Autodesk Inventor part; units mm, degrees
(part 4 of 4)
  line L1499 (-9.3571, 29.0765) -> (-9.424, 29.0765) construction
  spline S459 degree 2 poles (-9.424, 29.0765) (-9.4797, 29.0765) (-9.5645, 29.1568) (-9.5645, 29.2103) knots 0 0 0 1 2 2 2
  line L1500 (-9.424, 29.0765) -> (-9.4797, 29.0765) construction
  line L1501 (-9.4797, 29.0765) -> (-9.5645, 29.1568) construction
  line L1502 (-9.5645, 29.1568) -> (-9.5645, 29.2103) construction
  spline S460 degree 2 poles (-9.5645, 29.2103) (-9.5645, 29.2505) (-9.54, 29.2862) knots 0 0 0 1 1 1
  line L1503 (-9.5645, 29.2103) -> (-9.5645, 29.2505) construction
  line L1504 (-9.5645, 29.2505) -> (-9.54, 29.2862) construction
  line L1505 (-9.54, 29.2862) -> (-9.1385, 29.8883)
  spline S461 degree 2 poles (-9.1385, 29.8883) (-9.3392, 29.9218) (-9.4574, 30.0801) knots 0 0 0 1 1 1
  line L1506 (-9.1385, 29.8883) -> (-9.3392, 29.9218) construction
  line L1507 (-9.3392, 29.9218) -> (-9.4574, 30.0801) construction
  spline S462 degree 2 poles (-9.4574, 30.0801) (-9.5623, 30.2229) (-9.5623, 30.4147) knots 0 0 0 1 1 1
  line L1508 (-9.4574, 30.0801) -> (-9.5623, 30.2229) construction
  line L1509 (-9.5623, 30.2229) -> (-9.5623, 30.4147) construction
  spline S463 degree 2 poles (-9.5623, 30.4147) (-9.5623, 30.631) (-9.4284, 30.7804) knots 0 0 0 1 1 1
  line L1510 (-9.5623, 30.4147) -> (-9.5623, 30.631) construction
  line L1511 (-9.5623, 30.631) -> (-9.4284, 30.7804) construction
  spline S464 degree 2 poles (-9.4284, 30.7804) (-9.2812, 30.9477) (-9.0292, 30.9477) knots 0 0 0 1 1 1
  line L1512 (-9.4284, 30.7804) -> (-9.2812, 30.9477) construction
  line L1513 (-9.2812, 30.9477) -> (-9.0292, 30.9477) construction
  line L1514 (-9.0292, 30.9477) -> (-8.3624, 30.9477)
  spline S465 degree 2 poles (-8.3624, 30.9477) (-8.2285, 30.9477) (-8.2285, 30.8139) knots 0 0 0 1 1 1
  line L1515 (-8.3624, 30.9477) -> (-8.2285, 30.9477) construction
  line L1516 (-8.2285, 30.9477) -> (-8.2285, 30.8139) construction
  line L1517 (-8.2285, 30.8139) -> (-8.2285, 29.2126)
  spline S466 degree 2 poles (-8.2285, 29.2126) (-8.2285, 29.0787) (-8.3624, 29.0787) knots 0 0 0 1 1 1
  line L1518 (-8.2285, 29.2126) -> (-8.2285, 29.0787) construction
  line L1519 (-8.2285, 29.0787) -> (-8.3624, 29.0787) construction
  spline S467 degree 2 poles (-8.3624, 29.0787) (-8.4962, 29.0787) (-8.4962, 29.2126) knots 0 0 0 1 1 1
  line L1520 (-8.3624, 29.0787) -> (-8.4962, 29.0787) construction
  line L1521 (-8.4962, 29.0787) -> (-8.4962, 29.2126) construction
  spline S468 degree 2 poles (-7.1602, 29.8794) (-7.2941, 29.8794) (-7.2941, 30.0132) knots 0 0 0 1 1 1
  line L1522 (-7.1602, 29.8794) -> (-7.2941, 29.8794) construction
  line L1523 (-7.2941, 29.8794) -> (-7.2941, 30.0132) construction
  spline S469 degree 2 poles (-7.2941, 30.0132) (-7.2941, 30.147) (-7.1602, 30.147) knots 0 0 0 1 1 1
  line L1524 (-7.2941, 30.0132) -> (-7.2941, 30.147) construction
  line L1525 (-7.2941, 30.147) -> (-7.1602, 30.147) construction
  line L1526 (-7.1602, 30.147) -> (-7.0264, 30.147)
  spline S470 degree 2 poles (-7.0264, 30.147) (-6.9015, 30.147) (-6.8279, 30.2296) knots 0 0 0 1 1 1
  line L1527 (-7.0264, 30.147) -> (-6.9015, 30.147) construction
  line L1528 (-6.9015, 30.147) -> (-6.8279, 30.2296) construction
  spline S471 degree 2 poles (-6.8279, 30.2296) (-6.761, 30.3054) (-6.761, 30.4147) knots 0 0 0 1 1 1
  line L1529 (-6.8279, 30.2296) -> (-6.761, 30.3054) construction
  line L1530 (-6.761, 30.3054) -> (-6.761, 30.4147) construction
  spline S472 degree 2 poles (-6.761, 30.4147) (-6.761, 30.524) (-6.8279, 30.5976) knots 0 0 0 1 1 1
  line L1531 (-6.761, 30.4147) -> (-6.761, 30.524) construction
  line L1532 (-6.761, 30.524) -> (-6.8279, 30.5976) construction
  spline S473 degree 2 poles (-6.8279, 30.5976) (-6.9015, 30.6801) (-7.0287, 30.6801) knots 0 0 0 1 1 1
  line L1533 (-6.8279, 30.5976) -> (-6.9015, 30.6801) construction
  line L1534 (-6.9015, 30.6801) -> (-7.0287, 30.6801) construction
  line L1535 (-7.0287, 30.6801) -> (-7.1625, 30.6801)
  spline S474 degree 2 poles (-7.1625, 30.6801) (-7.3431, 30.6801) (-7.4814, 30.573) knots 0 0 0 1 1 1
  line L1536 (-7.1625, 30.6801) -> (-7.3431, 30.6801) construction
  line L1537 (-7.3431, 30.6801) -> (-7.4814, 30.573) construction
  spline S475 degree 2 poles (-7.4814, 30.573) (-7.5215, 30.544) (-7.5639, 30.544) knots 0 0 0 1 1 1
  line L1538 (-7.4814, 30.573) -> (-7.5215, 30.544) construction
  line L1539 (-7.5215, 30.544) -> (-7.5639, 30.544) construction
  spline S476 degree 2 poles (-7.5639, 30.544) (-7.6175, 30.544) (-7.6977, 30.6266) (-7.6977, 30.6823) knots 0 0 0 1 2 2 2
  line L1540 (-7.5639, 30.544) -> (-7.6175, 30.544) construction
  line L1541 (-7.6175, 30.544) -> (-7.6977, 30.6266) construction
  line L1542 (-7.6977, 30.6266) -> (-7.6977, 30.6823) construction
  spline S477 degree 2 poles (-7.6977, 30.6823) (-7.6977, 30.7448) (-7.642, 30.7871) knots 0 0 0 1 1 1
  line L1543 (-7.6977, 30.6823) -> (-7.6977, 30.7448) construction
  line L1544 (-7.6977, 30.7448) -> (-7.642, 30.7871) construction
  spline S478 degree 2 poles (-7.642, 30.7871) (-7.4346, 30.9477) (-7.1625, 30.9477) knots 0 0 0 1 1 1
  line L1545 (-7.642, 30.7871) -> (-7.4346, 30.9477) construction
  line L1546 (-7.4346, 30.9477) -> (-7.1625, 30.9477) construction
  line L1547 (-7.1625, 30.9477) -> (-7.0287, 30.9477)
  spline S479 degree 2 poles (-7.0287, 30.9477) (-6.7766, 30.9477) (-6.6272, 30.7827) knots 0 0 0 1 1 1
  line L1548 (-7.0287, 30.9477) -> (-6.7766, 30.9477) construction
  line L1549 (-6.7766, 30.9477) -> (-6.6272, 30.7827) construction
  spline S480 degree 2 poles (-6.6272, 30.7827) (-6.4934, 30.631) (-6.4934, 30.4147) knots 0 0 0 1 1 1
  line L1550 (-6.6272, 30.7827) -> (-6.4934, 30.631) construction
  line L1551 (-6.4934, 30.631) -> (-6.4934, 30.4147) construction
  spline S481 degree 2 poles (-6.4934, 30.4147) (-6.4934, 30.1671) (-6.6607, 30.0132) knots 0 0 0 1 1 1
  line L1552 (-6.4934, 30.4147) -> (-6.4934, 30.1671) construction
  line L1553 (-6.4934, 30.1671) -> (-6.6607, 30.0132) construction
  spline S482 degree 2 poles (-6.6607, 30.0132) (-6.4934, 29.8593) (-6.4934, 29.6118) knots 0 0 0 1 1 1
  line L1554 (-6.6607, 30.0132) -> (-6.4934, 29.8593) construction
  line L1555 (-6.4934, 29.8593) -> (-6.4934, 29.6118) construction
  spline S483 degree 2 poles (-6.4934, 29.6118) (-6.4934, 29.3932) (-6.6272, 29.2438) knots 0 0 0 1 1 1
  line L1556 (-6.4934, 29.6118) -> (-6.4934, 29.3932) construction
  line L1557 (-6.4934, 29.3932) -> (-6.6272, 29.2438) construction
  spline S484 degree 2 poles (-6.6272, 29.2438) (-6.7766, 29.0787) (-7.0287, 29.0787) knots 0 0 0 1 1 1
  line L1558 (-6.6272, 29.2438) -> (-6.7766, 29.0787) construction
  line L1559 (-6.7766, 29.0787) -> (-7.0287, 29.0787) construction
  line L1560 (-7.0287, 29.0787) -> (-7.1625, 29.0787)
  spline S485 degree 2 poles (-7.1625, 29.0787) (-7.4346, 29.0787) (-7.642, 29.2393) knots 0 0 0 1 1 1
  line L1561 (-7.1625, 29.0787) -> (-7.4346, 29.0787) construction
  line L1562 (-7.4346, 29.0787) -> (-7.642, 29.2393) construction
  spline S486 degree 2 poles (-7.642, 29.2393) (-7.6977, 29.2817) (-7.6977, 29.3441) knots 0 0 0 1 1 1
  line L1563 (-7.642, 29.2393) -> (-7.6977, 29.2817) construction
  line L1564 (-7.6977, 29.2817) -> (-7.6977, 29.3441) construction
  spline S487 degree 2 poles (-7.6977, 29.3441) (-7.6977, 29.3999) (-7.6175, 29.4824) (-7.5639, 29.4824) knots 0 0 0 1 2 2 2
  line L1565 (-7.6977, 29.3441) -> (-7.6977, 29.3999) construction
  line L1566 (-7.6977, 29.3999) -> (-7.6175, 29.4824) construction
  line L1567 (-7.6175, 29.4824) -> (-7.5639, 29.4824) construction
  spline S488 degree 2 poles (-7.5639, 29.4824) (-7.5215, 29.4824) (-7.4814, 29.4534) knots 0 0 0 1 1 1
  line L1568 (-7.5639, 29.4824) -> (-7.5215, 29.4824) construction
  line L1569 (-7.5215, 29.4824) -> (-7.4814, 29.4534) construction
  spline S489 degree 2 poles (-7.4814, 29.4534) (-7.3431, 29.3464) (-7.1625, 29.3464) knots 0 0 0 1 1 1
  line L1570 (-7.4814, 29.4534) -> (-7.3431, 29.3464) construction
  line L1571 (-7.3431, 29.3464) -> (-7.1625, 29.3464) construction
  line L1572 (-7.1625, 29.3464) -> (-7.0287, 29.3464)
  spline S490 degree 2 poles (-7.0287, 29.3464) (-6.9015, 29.3464) (-6.8279, 29.4311) knots 0 0 0 1 1 1
  line L1573 (-7.0287, 29.3464) -> (-6.9015, 29.3464) construction
  line L1574 (-6.9015, 29.3464) -> (-6.8279, 29.4311) construction
  spline S491 degree 2 poles (-6.8279, 29.4311) (-6.761, 29.5069) (-6.761, 29.6162) knots 0 0 0 1 1 1
  line L1575 (-6.8279, 29.4311) -> (-6.761, 29.5069) construction
  line L1576 (-6.761, 29.5069) -> (-6.761, 29.6162) construction
  spline S492 degree 2 poles (-6.761, 29.6162) (-6.761, 29.8549) (-6.993, 29.8794) knots 0 0 0 1 1 1
  line L1577 (-6.761, 29.6162) -> (-6.761, 29.8549) construction
  line L1578 (-6.761, 29.8549) -> (-6.993, 29.8794) construction
  line L1579 (-6.993, 29.8794) -> (-7.1602, 29.8794)
  circle A34 centre (12.0262, -0.3274) radius 1.5
  circle A35 centre (7.9565, 12.6117) radius 1.5
  circle A36 centre (-5.5726, 40.6117) radius 1.5
  circle A37 centre (5.1417, 40.6117) radius 1.5
  circle A38 centre (2.0046, 47.4047) radius 1.5
  circle A39 centre (-7.8666, -21.4194) radius 1.5
  circle A40 centre (11.3019, -20.7894) radius 1.5
  circle A41 centre (0.0461, -47.8325) radius 0.9643
  circle A42 centre (3.801, -45.6645) radius 0.9643
  circle A43 centre (-3.7089, -50.0004) radius 0.9643
  circle A44 centre (-2.9194, -17.7327) radius 1.5
  circle A45 centre (7.523, 47.4047) radius 1.5
  circle A46 centre (5.1417, 36.8617) radius 1.5
  circle A47 centre (-5.5726, 36.8617) radius 1.5
  circle A48 centre (12.0262, -5.6846) radius 1.5
  circle A49 centre (-2.4381, -5.6846) radius 1.5
  circle A50 centre (3.6975, 10.0791) radius 1.5
  circle A51 centre (-10.9297, 36.8617) radius 1.5
  circle A52 centre (-0.2154, 36.8617) radius 1.5
  circle A53 centre (11.5703, 36.8617) radius 1.5
  circle A54 centre (-7.8666, -17.7327) radius 1.5
  circle A55 centre (11.3019, -16.6927) radius 1.5
  circle A56 centre (-3.7089, -45.6645) radius 0.9643
  circle A57 centre (3.801, -50.0004) radius 0.9643
  circle A58 centre (0.0461, -52.1683) radius 0.9643
  circle A59 centre (0.0461, -43.4966) radius 0.9643
  circle A60 centre (-2.9194, -21.4194) radius 1.5
  circle A61 centre (12.6945, 47.4047) radius 1.5
  circle A62 centre (11.5703, 40.6117) radius 1.5
  circle A63 centre (-0.2154, 40.6117) radius 1.5
  circle A64 centre (-10.9297, 40.6117) radius 1.5
  circle A65 centre (0.1842, 12.6117) radius 1.5
  circle A66 centre (-2.4381, -0.3274) radius 1.5
  circle A67 centre (16.6071, -57.5893) radius 0.8036
  circle A68 centre (-16.6071, -57.5893) radius 0.8036
  circle A69 centre (16.6071, 57.5893) radius 0.8036
  circle A70 centre (-16.6071, 57.5893) radius 0.8036
  line L1580 (-16.6071, -7.9473) -> (-9.0292, -7.9473)
  line L1581 (-9.0292, -7.9473) -> (-9.0292, -14.8361)
  line L1582 (-9.0292, -14.8361) -> (-16.6071, -14.8361)
  line L1583 (-16.6071, -14.8361) -> (-16.6071, -7.9473)
  line L1584 (1.2846, -7.9473) -> (3.801, -7.9473)
  line L1585 (3.801, -7.9473) -> (3.801, -14.8361)
  line L1586 (3.801, -14.8361) -> (1.2846, -14.8361)
  line L1587 (1.2846, -14.8361) -> (1.2846, -7.9473)
  line L1588 (6.023, 5.9584) -> (9.8019, 5.9584)
  line L1589 (9.8019, 5.9584) -> (9.8019, 1.1726)
  line L1590 (9.8019, 1.1726) -> (6.023, 1.1726)
  line L1591 (6.023, 1.1726) -> (6.023, 5.9584)
  line L1592 (-9.0292, -7.9473) -> (-4.6732, -7.9473)
  line L1593 (-4.6732, -7.9473) -> (-4.6732, 2.6847)
  line L1594 (-4.6732, 2.6847) -> (-2.4381, 2.6847)
  line L1595 (-2.4381, 2.6847) -> (-2.4381, 14.2993)
  line L1596 (-2.4381, 14.2993) -> (-2.4381, 15.7273)
  line L1597 (-2.4381, 15.7273) -> (12.0262, 15.7273)
  line L1598 (12.0262, 15.7273) -> (12.0262, 2.5813)
  line L1599 (12.0262, 2.5813) -> (14.5265, 2.5813)
  line L1600 (14.5265, 2.5813) -> (14.5265, -12.7047)
  line L1601 (14.5265, -12.7047) -> (14.5265, -23.4688)
  line L1602 (14.5265, -23.4688) -> (-10.9297, -23.4688)
  line L1603 (-10.9297, -23.4688) -> (-10.9297, -14.8361)
  point P0 (0, 0)
  dimension "d0" = 3
  dimension "d1" = 3
  dimension "d2" = 3
  dimension "d3" = 3
  dimension "d4" = 3
  dimension "d5" = 3
  constraints: 892 end point, 71 centre point, 64 point on circle, 11 perpendicular, 6 parallel, 5 horizontal, 2 vertical, 1 point on line, 1479 other
  measures "d0" diameter of A65
  measures "d1" diameter of A50
  measures "d2" diameter of A35
  measures "d3" diameter of A66
  measures "d4" diameter of A44
  measures "d5" diameter of A55
extrude "Выдавливание1" add sketch "Эскиз1" along normal blind 2 contours L1580 L1581 L1582 L1583 | L1592 L1593 L1594 L1595 L1596 L1597 L1598 L1599 L1600 L1601 L1602 L1603 L1582 L1581 | L1584 L1585 L1586 L1587 | L1588 L1589 L1590 L1591
extrude "Выдавливание2" add sketch "Эскиз1" against normal blind 8 contours L1580 L1581 L1582 L1583 | L1584 L1585 L1586 L1587 | L1588 L1589 L1590 L1591
